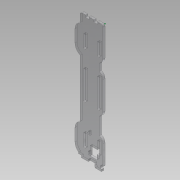
# Autodesk Inventor part: Left_wall
Saved by Autodesk Inventor 2016 (Build 200138000, 138)
## iProperties
Created: 2015-06-19
Part Number: Left_wall
Material: Generic
Document SubType Name: Modeling
Designer: Openlab
Density: 1 g/cm^3
Appearance: Polycarbonate - Clear
Author: Openlab
Autodesk Inventor part; units mm, degrees
ref_plane "YZ Plane" through (0, 0, 0) normal (1, 0, 0) x (0, 1, 0)
ref_plane "XZ Plane" through (0, 0, 0) normal (0, 1, 0) x (-1, 0, 0)
ref_plane "XY Plane" through (0, 0, 0) normal (0, 0, 1) x (1, 0, 0)
sketch "Sketch1" plane through (0, 0, 0) normal (0, 1, 0) x (-1, 0, 0)
  line L0 (28, -25) -> (25, -25)
  line L1 (28, -43) -> (25, -43)
  line L2 (28, -68.5) -> (25, -68.5)
  line L3 (28, -109.5) -> (25, -109.5)
  line L4 (8, -68.5) -> (5, -68.5)
  line L5 (8, -109.5) -> (5, -109.5)
  line L6 (8, -43) -> (5, -43)
  line L7 (8, -25) -> (5, -25)
  line L8 (25, -109.5) -> (25, -68.5)
  line L9 (25, -43) -> (25, -25)
  line L10 (8, -109.5) -> (8, -68.5)
  line L11 (8, -43) -> (8, -25)
  line L12 (8, -160.5) -> (8, -149)
  line L13 (28, -149) -> (25, -149)
  line L14 (8, -149) -> (5, -149)
  line L15 (25, -149) -> (25, -167)
  line L16 (25, -167) -> (28, -167)
  line L17 (5, -167) -> (8.5, -167)
  line L18 (21.5, -169) -> (19.7, -169)
  line L19 (19.7, -169) -> (19.7, -174)
  line L20 (19.7, -174) -> (21.5, -174)
  line L21 (21.5, -174) -> (21.5, -169)
  line L22 (16.5, -110.2512) -> (16.5, -143.2512) construction
  line L23 (28, -25) -> (28, -43)
  line L24 (28, -68.5) -> (28, -109.5)
  line L25 (28, -149) -> (28, -167)
  line L26 (5, -167) -> (5, -149)
  line L27 (5, -109.5) -> (5, -68.5)
  line L28 (5, -43) -> (5, -25)
  line L29 (13, -3) -> (8, -3)
  line L30 (20, -3) -> (20, 0)
  line L31 (20, 0) -> (13, 0)
  line L32 (13, 0) -> (13, -3)
  line L33 (20, -3) -> (25, -3)
  line L34 (4.25, -179) -> (4.25, -182)
  line L35 (11.75, -179) -> (21.25, -179)
  line L36 (21.25, -179) -> (21.25, -182)
  line L37 (21.25, -182) -> (31.0828, -182)
  line L38 (31.25, -179) -> (33, -179)
  line L39 (4.25, -182) -> (2.25, -182)
  line L40 (25, -3) -> (25, 0)
  line L41 (25, 0) -> (30, 0)
  line L42 (8, -3) -> (8, 0)
  line L43 (8, 0) -> (3, 0)
  line L44 (2.25, -185) -> (11.2894, -185)
  arc A0 (31.0828, -182) -> (31.25, -179) centre (4.25, -179) ccw
  arc A1 (5, -141.5838) -> (0, -149) centre (8, -149) ccw
  arc A2 (5, -61.0838) -> (0, -68.5) centre (8, -68.5) ccw
  line L45 (5, -50.4162) -> (5, -61.0838)
  line L46 (5, -116.9162) -> (5, -141.5838)
  line L47 (19.5, -129.25) -> (13.2, -129.25) construction
  arc A3 (0, -109.5) -> (5, -116.9162) centre (8, -109.5) ccw
  line L48 (0, -177.7474) -> (0, -149)
  arc A4 (0, -43) -> (5, -50.4162) centre (8, -43) ccw
  line L49 (0, -109.5) -> (0, -68.5)
  line L50 (0, -43) -> (0, -3)
  arc A5 (33, -54.4564) -> (40.5, -43) centre (28, -43) ccw
  line L51 (40.5, -25) -> (40.5, -43)
  arc A6 (40.5, -25) -> (33, -13.5436) centre (28, -25) ccw
  line L52 (33, -3) -> (33, -13.5436)
  arc A7 (40.5, -149) -> (33, -137.5436) centre (28, -149) ccw
  line L53 (40.5, -167) -> (40.5, -149)
  arc A8 (35.5, -177) -> (40.5, -167) centre (28, -167) ccw
  line L54 (33, -54.4564) -> (33, -137.5436)
  arc A9 (33, -3) -> (30, 0) centre (30, -3) ccw
  arc A10 (3, 0) -> (0, -3) centre (3, -3) ccw
  line L55 (21.5, -144) -> (19.7, -144)
  line L56 (19.7, -144) -> (19.7, -149)
  line L57 (19.7, -149) -> (21.5, -149)
  line L58 (21.5, -149) -> (21.5, -144)
  line L59 (18.5, -160.5) -> (8.5, -160.5)
  line L60 (8.5, -167) -> (8.5, -173.5)
  line L61 (8.5, -173.5) -> (18.5, -173.5)
  line L62 (18.5, -173.5) -> (18.5, -160.5)
  line L63 (13.5, -163.9683) -> (13.5, -168.686) construction
  line L64 (14.8699, -167) -> (11.7199, -167) construction
  arc A11 (11.2894, -185) -> (11.75, -182) centre (1.75, -182) ccw
  line L65 (11.75, -182) -> (11.75, -179)
  line L66 (14.25, -179) -> (14.25, -182) construction
  line L67 (14.25, -182) -> (4.25, -182) construction
  line L68 (31.25, -179) -> (31.25, -182) construction
  line L69 (31.25, -182) -> (31.0828, -182) construction
  line L70 (33, -179) -> (35.5, -179)
  line L71 (35.5, -179) -> (35.5, -177)
  line L72 (33, -179) -> (33, -174.1753) construction
  line L73 (28, -179) -> (28, -186) construction
  line L74 (28, -186) -> (25, -186) construction
  line L75 (25, -186) -> (25, -179) construction
  line L76 (31.25, -179) -> (21.25, -179) construction
  line L77 (4.25, -179) -> (0, -177.7474)
  line L78 (1.75, -182.5) -> (1.75, -184.5)
  arc A12 (2.25, -182) -> (1.75, -182.5) centre (2.25, -182.5) ccw
  arc A13 (1.75, -184.5) -> (2.25, -185) centre (2.25, -184.5) ccw
  line L79 (8.5, -160.5) -> (8, -160.5)
  line L80 (26.5, -73.5989) -> (26.5, -105.0523) construction
  line L81 (6.5, -72.0232) -> (6.5, -105.7187) construction
  point P0 (0, 0)
  point P1 (1.75, -185)
  dimension "d7" = 18
  dimension "d8" = 25.5
  dimension "d9" = 41
  dimension "d39" = 18
  dimension "d45" = 5
  dimension "d56" = 3
  dimension "d61" = 39.5
  dimension "d64" = 12
  dimension "d65" = 7
  dimension "d74" = 176
  dimension "d75" = 17
  dimension "d85" = 10
  dimension "d90" = 5
  dimension "d92" = 25
  dimension "d104" = 6
  dimension "d105" = 5
  dimension "d106" = 1.8
  dimension "d107" = 3.5
  dimension "d108" = 20
  dimension "d112" = 8
  dimension "d113" = 12
  dimension "d114" = 7
  dimension "d115" = 10
  dimension "d116" = 3
  dimension "d121" = 2.5
  dimension "d122" = 25
  dimension "d123" = 7
  dimension "d124" = 10
  dimension "d125" = 2.5
  dimension "d126" = 2.5
  dimension "d127" = 0.5
  dimension "d129" = 13
  dimension "d130" = 10
  dimension "d134" = 17
  constraints: 165 end point, 28 point on circle, 26 collinear, 23 tangent, 21 point on line, 16 perpendicular, 15 vertical, 14 centre point, 8 equal length, 8 horizontal, 8 parallel, 7 coincident, 5 equal radius, 10 other
  measures "d7" distance between parallel lines of L1 L0
  measures "d8" distance between parallel lines of L2 L1
  measures "d9" distance between parallel lines of L3 L2
  measures "d39" distance of L13.end L15.end
  measures "d45" distance of L20.end L18.start
  measures "d56" distance of L0.start L0.end
  measures "d61" distance between parallel lines of L3 L13
  measures "d64" distance between parallel lines of L16 L38
  measures "d65" distance of L30.end L31.end
  measures "d74" distance between parallel lines of L38 L33
  measures "d75" distance between parallel lines of L42 L40
  measures "d85" distance from line of L38.start L36
  measures "d90" distance between parallel lines of L48 L26
  measures "d92" diameter of A5
  measures "d104" diameter of A9
  measures "d105" distance between parallel lines of L20 L35
  measures "d106" distance of L55.start L55.end
  measures "d107" distance between parallel lines of L58 L15
  measures "d108" distance between parallel lines of L18 L57
  measures "d112" distance between parallel lines of L63 L21
  measures "d113" distance between parallel lines of L35 L64
  measures "d114" distance between parallel lines of L66 L36
  measures "d115" distance between parallel lines of L34 L66
  measures "d116" distance between parallel lines of L39 L44
  measures "d121" distance of L38.end L70.end
  measures "d122" distance between parallel lines of L0 L41
  measures "d123" distance of L73.start L73.end
  measures "d124" distance between parallel lines of L78 L65
  measures "d125" distance between parallel lines of L65 L66
  measures "d126" distance of L34.end point (1.75, -182)
  measures "d127" radius of A12
  measures "d129" distance between parallel lines of L61 L59
  measures "d130" distance of L60.end L61.end
  measures "d134" distance between parallel lines of L10 L8
extrude "Extrusion3" add sketch "Sketch1" along normal blind 3
body "Solid3"
